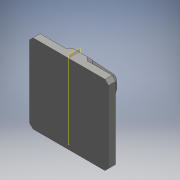
# Autodesk Inventor part: TrackPivotConnector
Saved by Autodesk Inventor 2016 (Build 200138000, 138)
## iProperties
Created: 2016-11-02
Part Number: TrackPivotConnector
Material: Generic
Document SubType Name: Modeling
Designer: mattc
Density: 1 g/cm^3
Appearance: Smooth - Medium Gray
Author: mattc
Autodesk Inventor part; units mm, degrees
ref_plane "YZ Plane" through (0, 0, 0) normal (1, 0, 0) x (0, 1, 0)
ref_plane "XZ Plane" through (0, 0, 0) normal (0, 1, 0) x (-1, 0, 0)
ref_plane "XY Plane" through (0, 0, 0) normal (0, 0, 1) x (1, 0, 0)
sketch "Sketch1" plane through (0, 0, 0) normal (0, 1, 0) x (-1, 0, 0)
  line L0 (0, 0) -> (22.3, 0)
  line L1 (22.3, 0) -> (22.3, -22.3)
  line L2 (22.3, -22.3) -> (0, -22.3)
  line L3 (0, -22.3) -> (0, 0)
  dimension "d0" = 22.3
  dimension "d1" = 22.3
  constraints: 8 end point, 2 parallel, 1 horizontal, 1 perpendicular
  measures "d0" distance of L1.end L2.end
  measures "d1" distance of L0.end L1.end
extrude "Extrusion1" add sketch "Sketch1" along normal blind 3
ref_plane "Work Plane1" through (-11.15, 0, 0) normal (1, 0, 0) x (0, 0, -1)
sketch "Sketch3" plane through (-11.15, 0, 0) normal (1, 0, 0) x (0, 0, -1)
  line L0 (0, 3) -> (22.3, 3) projected
  circle A0 centre (11.15, 8) radius 2.5
  arc A1 (13.8913, 10.913) -> (8.4087, 10.913) centre (11.15, 8) ccw
  line L1 (0, 0) -> (0, 3) projected
  line L2 (0, 3) -> (8.4087, 10.913)
  line L3 (13.8913, 10.913) -> (22.3, 3)
  dimension "d5" = 5
  dimension "d6" = 8
  dimension "d7" = 11.15
  dimension "d8" = 5
  constraints: 4 end point, 2 centre point, 2 point on circle, 2 tangent, 1 coincident
  measures "d5" diameter of A0
  measures "d6" diameter of A1
  measures "d7" distance from line of A0.centre L1
  measures "d8" distance from line of L0 A0.centre
extrude "Extrusion2" add sketch "Sketch3" along normal mid plane 5
chamfer "Chamfer1" distance 1 angle 45 1 edges at (-8.65, 3, -11.15)
chamfer "Chamfer2" distance 1 angle 45 1 edges at (-13.65, 3, -11.15)
chamfer "Chamfer3" distance 1 angle 45 3 edges at (-13.65, 12, -11.15) (-13.65, 7.4565, -17.5643) (-13.65, 7.4565, -4.7357)
chamfer "Chamfer4" distance 1 angle 45 3 edges at (-8.65, 7.4565, -4.7357) (-8.65, 12, -11.15) (-8.65, 7.4565, -17.5643)
chamfer "Chamfer5" distance 1 angle 45 10 edges at (-18.475, 3, 0) (-22.3, 3, -11.15) (-3.825, 3, 0) (0, 3, -11.15) (-3.825, 3, -22.3) (-18.475, 3, -22.3) (0, 1.5, -22.3) (0, 1.5, 0) (-22.3, 1.5, -22.3) (-22.3, 1.5, 0)
chamfer "Chamfer6" distance 1 angle 45 2 edges at (-7.15, 2.5, 0) (-15.15, 2.5, 0)
chamfer "Chamfer7" distance 1 angle 45 2 edges at (-7.15, 2.5, -22.3) (-15.15, 2.5, -22.3)
equation "\"d1\" = d0"
equation "\"d7\" = 0.5 * d0"
equation "\"d4\" = -0.5 * d0"
body "Solid1"
